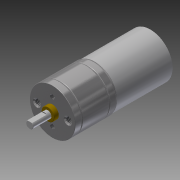
# Autodesk Inventor part: motor_dc
Saved by Autodesk Inventor 2015 (Build 190159000, 159)
## iProperties
Created: 2015-03-18
Part Number: motor_dc
Material: Ogólny
Document SubType Name: Modeling
Designer: Marcin
Density: 1 g/cm^3
Appearance: Galwanizowana
Author: Marcin
Autodesk Inventor part; units mm, degrees
ref_plane "YZ Plane" through (0, 0, 0) normal (1, 0, 0) x (0, 1, 0)
ref_plane "XZ Plane" through (0, 0, 0) normal (0, 1, 0) x (-1, 0, 0)
ref_plane "XY Plane" through (0, 0, 0) normal (0, 0, 1) x (1, 0, 0)
sketch "Szkic1" plane through (0, 0, 0) normal (0, 0, 1) x (1, 0, 0)
  circle A0 centre (0, 0) radius 12.5
  dimension "d0" = 25
  constraints: 1 centre point, 1 coincident
  measures "d0" diameter of A0
extrude "Wyciągnięcie proste1" add sketch "Szkic1" along normal blind 4
sketch "Szkic2" plane through (0, 0, 0) normal (0, 0, -1) x (-1, 0, 0)
  circle A0 centre (0, 0) radius 12.5 projected
fillet "Zaokrąglenie1" radius 0.5 1 edges at (-12.5, 0, 0)
extrude "Wyciągnięcie proste2" add sketch "Szkic2" along normal blind 15
fillet "Zaokrąglenie2" radius 0.5 1 edges at (12.5, 0, 0)
fillet "Zaokrąglenie3" radius 0.5 1 edges at (12.5, 0, -15)
sketch "Szkic4" plane through (0, 0, -15) normal (0, 0, -1) x (-1, 0, 0)
  circle A0 centre (0, 0) radius 12.5 projected
extrude "Wyciągnięcie proste3" add sketch "Szkic4" along normal blind 4
fillet "Zaokrąglenie4" radius 0.5 1 edges at (12.5, 0, -15)
sketch "Szkic5" plane through (0, 0, 4) normal (0, 0, 1) x (1, 0, 0)
  circle A0 centre (0, 0) radius 3.5
  dimension "d11" = 7
  constraints: 1 centre point, 1 coincident
  measures "d11" diameter of A0
extrude "Wyciągnięcie proste4" add sketch "Szkic5" along normal blind 2.5
sketch "Szkic6" plane through (0, 0, 6.5) normal (0, 0, 1) x (1, 0, 0)
  circle A0 centre (0, 0) radius 2
  dimension "d14" = 4
  constraints: 1 centre point, 1 coincident
  measures "d14" diameter of A0
extrude "Wyciągnięcie proste5" add sketch "Szkic6" along normal blind 10
sketch "Szkic7" plane through (0, 0, 16.5) normal (0, 0, 1) x (1, 0, 0)
  circle A0 centre (0, 0) radius 2 projected
  circle A1 centre (0, 0) radius 2 projected
  line L0 (1.3229, 1.5) -> (1.3229, 1.5)
  line L1 (-3.3787, -2) -> (2.8088, -2) construction
  circle A2 centre (0, 0) radius 2
  line L2 (1.3229, 1.5) -> (-1.3229, 1.5)
  dimension "d17" = 3.5
  constraints: 6 end point, 5 point on circle, 3 horizontal, 1 coincident, 1 tangent, 3 other
  measures "d17" distance between parallel lines of L1 L0
extrude "Wyciągnięcie proste6" cut sketch "Szkic7" against normal blind 8 contours L2 A0 picked at (-0.3089, 1.5908)
fillet "Zaokrąglenie5" radius 0.25 1 edges at (-12.5, 0, 4)
fillet "Zaokrąglenie6" radius 0.25 3 edges at (-3.5, 0, 6.5) (-0.8229, -1.8229, 16.5) (1.8229, 0.8229, 16.5)
sketch "Szkic8" plane through (0, 0, -19) normal (0, 0, -1) x (-1, 0, 0)
  circle A0 centre (0, 0) radius 12.2
  dimension "d22" = 24.4
  constraints: 1 centre point, 1 coincident
  measures "d22" diameter of A0
extrude "Wyciągnięcie proste7" add sketch "Szkic8" along normal blind 30.8
sketch "Szkic9" plane through (0, 0, 4) normal (0, 0, 1) x (1, 0, 0)
  circle A0 centre (0, 0) radius 3.5 projected
  circle A1 centre (0, 0) radius 12.25 projected
  line L0 (0, 12.25) -> (0, -12.25) construction
  line L1 (-10.7735, 0) -> (10.2994, 0) construction
  point P0 (0, 7)
  point P1 (0, -7)
  dimension "d25" = 14
  constraints: 4 end point, 3 point on line, 2 midpoint, 2 point on circle, 1 horizontal, 1 symmetric about line, 1 vertical
  measures "d25" distance of point (0, 7) point (0, -7)
hole "Otwór1" at (0, 7, 4) at (0, -7, 4) direction (0, 0, -1) diameter 2.459 depth 6 tip angle 118 thread size "M3x0.5" class "6H" standard "ISO Metric profile"
sketch "Szkic10" plane through (0, 0, 4) normal (0, 0, 1) x (1, 0, 0)
  circle A0 centre (0, 0) radius 12.25 projected
  circle A1 centre (0, 7) radius 1.2295 construction
  circle A2 centre (0, -7) radius 1.2295 construction
  line L0 (0, 7) -> (0, -7) construction
  line L1 (-8.5, 0) -> (7.3075, 0) construction
  point P0 (8.5, 0)
  point P1 (0, 0)
  dimension "d33" = 17
  constraints: 4 end point, 1 horizontal, 1 midpoint, 1 point on line, 1 symmetric about line, 1 vertical
  measures "d33" distance of point (8.5, 0) L1.start
hole "Otwór2" at (-8.5, 0, 4) at (8.5, 0, 4) direction (0, 0, -1) diameter 3.242 depth 11.8 tip angle 118 countersink diameter 4.5 countersink angle 90 thread size "M4x0.7" class "6H" standard "ANSI Metric M Profile"
fillet "Zaokrąglenie7" radius 1 1 edges at (12.5, 0, -19)
fillet "Zaokrąglenie8" radius 1 1 edges at (12.2, 0, -19)
